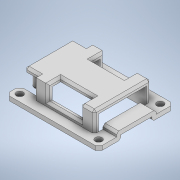
# Autodesk Inventor part: motor holder top
Saved by Autodesk Inventor 2022 (Build 260153000, 153)
## iProperties
Created: 2021-11-29
Part Number: motor holder top
Material: Generic
Document SubType Name: Modeling
Designer: Alec Warren
Density: 1 g/cm^3
Appearance: Default
Author: Alec Warren
Autodesk Inventor part; units mm, degrees
ref_plane "YZ Plane" through (0, 0, 0) normal (1, 0, 0) x (0, 1, 0)
ref_plane "XZ Plane" through (0, 0, 0) normal (0, 1, 0) x (-1, 0, 0)
ref_plane "XY Plane" through (0, 0, 0) normal (0, 0, 1) x (1, 0, 0)
sketch "Sketch1" plane through (0, 0, 0) normal (0, 1, 0) x (-1, 0, 0)
  line L0 (0, 0) -> (0, 22.5)
  line L1 (-41.8, 0) -> (0, 0)
  line L2 (0, 11.25) -> (-37, 11.25)
  line L3 (-39.4, 11.25) -> (-25.4, 11.25)
  line L4 (-25.4, 11.25) -> (-14.15, 11.25)
  line L5 (-14.15, 11.25) -> (-5.55, 11.25)
  line L6 (-5.55, 11.25) -> (-5.55, 2.45)
  line L7 (-5.55, 11.25) -> (-5.55, 20.05)
  circle A0 centre (-5.55, 2.45) radius 1.375
  circle A1 centre (-5.55, 20.05) radius 1.375
  line L8 (-37, 0) -> (-37, 22.5)
  line L9 (0, 22.5) -> (0, 28.9)
  line L10 (0, 0) -> (0, -6.4)
  line L11 (0, -6.4) -> (-41.8, -6.4)
  line L12 (-41.8, 28.9) -> (0, 28.9)
  line L13 (0, -3.2) -> (-3.2, -3.2)
  line L14 (0, 25.7) -> (-3.2, 25.7)
  circle A2 centre (-3.2, -3.2) radius 1.6
  circle A3 centre (-40.2, -3.2) radius 1.6
  circle A4 centre (-3.2, 25.7) radius 1.6
  circle A5 centre (-3.2, 25.7) radius 1.6
  circle A6 centre (-40.2, 25.7) radius 1.6
  line L15 (-5.55, 0) -> (-2.35, 0)
  line L16 (-5.55, 0) -> (-8.75, 0)
  line L17 (-2.35, 0) -> (-8.75, 0)
  line L18 (-8.75, 0) -> (-8.75, 22.5)
  line L19 (-8.75, 22.5) -> (-2.35, 22.5)
  line L20 (-2.35, 22.5) -> (-2.35, 0)
  line L21 (-37, 11.25) -> (-30.6, 11.25)
  line L22 (-30.6, 22.5) -> (-30.6, 0)
  line L23 (-37, 22.5) -> (-37, 28.9)
  line L24 (-30.6, 22.5) -> (-30.6, 28.9)
  line L25 (-30.6, 0) -> (-30.6, -6.4)
  line L26 (-37, -6.4) -> (-37, 0)
  line L27 (-8.75, 0) -> (-8.75, -6.4)
  line L28 (-8.75, 22.5) -> (-8.75, 28.9)
  line L29 (-37, 28.9) -> (-43.4, 28.9)
  line L30 (-43.4, 28.9) -> (-43.4, -6.4)
  line L31 (-43.4, -6.4) -> (-37, -6.4)
  line L32 (-8.75, 28.9) -> (-15.15, 28.9)
  line L33 (-15.15, 28.9) -> (-15.15, -6.4)
  line L34 (-30.6, 11.25) -> (-30.6, 22.5)
  line L35 (-30.6, 16.875) -> (-30.6, 18.475)
  line L36 (-30.6, 16.875) -> (-30.6, 15.275)
  line L37 (-30.6, 18.475) -> (-15.15, 18.475)
  line L38 (-15.15, 18.475) -> (-15.15, 15.275)
  line L39 (-30.6, 15.275) -> (-30.6, 18.475)
  line L40 (-43.4, 11.25) -> (-37, 11.25)
  line L41 (-30.6, 11.25) -> (-30.6, 0)
  line L42 (-30.6, 5.625) -> (-30.6, 4.025)
  line L43 (-30.6, 4.025) -> (-15.15, 4.025)
  line L44 (-37, 0) -> (-43.4, 0)
  line L45 (0, 28.9) -> (0, 22.5)
  line L46 (0, 22.5) -> (-43.4, 22.5)
  line L47 (0, 0) -> (-43.4, 0)
  line L48 (-37, 22.5) -> (-30.6, 22.5)
  line L49 (-30.6, 22.5) -> (-30.6, 24.5)
  line L50 (-30.6, 24.5) -> (-37, 24.5)
  line L51 (-37, 24.5) -> (-37, 22.5)
  line L52 (-37, 0) -> (-30.6, 0)
  line L53 (-30.6, 0) -> (-30.6, -2)
  line L54 (-30.6, -2) -> (-37, -2)
  line L55 (-37, -2) -> (-37, 0)
  line L56 (-15.15, 22.5) -> (-8.75, 22.5)
  line L57 (-8.75, 22.5) -> (-8.75, 24.5)
  line L58 (-8.75, 24.5) -> (-15.15, 24.5)
  line L59 (-15.15, 24.5) -> (-15.15, 22.5)
  line L60 (-15.15, 0) -> (-8.75, 0)
  line L61 (-8.75, 0) -> (-8.75, -2)
  line L62 (-8.75, -2) -> (-15.15, -2)
  line L63 (-15.15, -2) -> (-15.15, 0)
  line L64 (-30.6, 24.5) -> (-15.15, 24.5)
  line L65 (-15.15, -2) -> (-30.6, -2)
  line L66 (-37, 22.5) -> (-37, 18.5)
  line L67 (-37, 18.5) -> (-43.4, 18.5)
  line L68 (-37, 0) -> (-37, 4)
  line L69 (-37, 4) -> (-43.4, 4)
  line L70 (-43.4, 20.5) -> (-37, 20.5)
  line L71 (-37, 2) -> (-43.4, 2)
  point P0 (-15.15, 0)
  dimension "d0" = 22.5
  dimension "d2" = 37
  dimension "d4" = 14
  dimension "d5" = 11.25
  dimension "d6" = 8.6
  dimension "d7" = 8.8
  dimension "d8" = 8.8
  dimension "d9" = 2.75
  dimension "d10" = 2.75
  dimension "d12" = 6.4
  dimension "d13" = 6.4
  dimension "d18" = 3.2
  dimension "d22" = 3.2
  dimension "d39" = 3.2
  dimension "d40" = 3.2
  dimension "d41" = 6.4
  dimension "d42" = 6.4
  dimension "d43" = 6.4
  dimension "d44" = 1.6
  dimension "d45" = 1.6
  dimension "d46" = 1.6
  dimension "d47" = 2
  dimension "d48" = 2
  dimension "d49" = 2
  dimension "d50" = 2
  dimension "d57" = 4
  dimension "d58" = 4
  constraints: 142 end point, 37 point on line, 16 horizontal, 15 perpendicular, 14 parallel, 7 centre point, 7 midpoint, 5 collinear, 4 coincident, 4 vertical, 2 symmetric about line, 1 equal radius, 12 other
  measures "d0" distance of L0.start L0.end
  measures "d2" distance of L2.start L2.end
  measures "d4" distance of L3.start L3.end
  measures "d5" distance of L3.end L4.end
  measures "d6" distance of L4.end L5.end
  measures "d7" distance of L5.end L6.end
  measures "d8" distance of L5.end L7.end
  measures "d9" diameter of A0
  measures "d10" diameter of A1
  measures "d12" distance of L0.end L9.end
  measures "d13" distance of L0.start L10.end
  measures "d18" distance of L14.start L14.end
  measures "d22" diameter of A4
  measures "d39" distance of L15.start L15.end
  measures "d40" distance of L15.start L16.end
  measures "d41" distance of L2.end L21.end
  measures "d42" distance of L23.end L29.end
  measures "d43" distance of L28.end L32.end
  measures "d44" distance of L35.start L35.end
  measures "d45" distance of L35.start L36.end
  measures "d46" distance of L42.start L42.end
  measures "d47" distance of L49.end L48.end
  measures "d48" distance of L52.end L53.end
  measures "d49" distance of L57.end L56.end
  measures "d50" distance of L60.end L61.end
  measures "d57" distance of L8.end L66.end
  measures "d58" distance of L8.start L68.end
extrude "Extrusion1" add sketch "Sketch1" along normal blind 2 contours L10 L11 L27 L1 | L46 L19 L28 L12 L9 | L27 L62 L33 L1 | L11 L33 L62 L27 | L46 L33 L58 L28 | L33 L65 L25 L1 | L11 L25 L65 L33 | L28 L58 L33 L12 | L46 L24 L64 L33 | L25 L54 L26 L1 | L11 L26 L54 L25 | L33 L64 L24 L12 | L46 L23 L50 L24 | L26 L11 L31 L30 L44 L1 | L1 L44 L30 L71 L8 | L24 L50 L23 L12 | L46 L30 L29 L12 L23 | L8 L70 L30 L46 | L71 L30 L69 L8 | L8 L67 L30 L70
extrude "Extrusion5" add sketch "Sketch1" along normal blind 2 from surface at 2 contours L71 L30 L69 L8 | L8 L67 L30 L70 | L69 L30 L40 L3 L8 | L8 L3 L40 L30 L67
extrude "Extrusion6" add sketch "Sketch1" along normal blind 7.3 from surface at 2 contours L27 L62 L33 L1 | L46 L33 L58 L28 | L25 L54 L26 L1 | L46 L23 L50 L24
extrude "Extrusion7" add sketch "Sketch1" along normal blind 2 from surface at 9.3 contours L1 L18 L2 L20 | L2 L18 L19 L20 | L27 L62 L33 L1 | L1 L33 L2 L18 | L46 L33 L58 L28 | L18 L2 L33 L46 | L25 L54 L26 L1 | L1 L8 L2 L22 | L43 L22 L2 L33 | L33 L2 L22 L37 | L46 L23 L50 L24 | L22 L2 L8 L46 | A0 | A1
chamfer "Chamfer2" distance 1 angle 45 4 edges at (40.2, 0, 18.5) (40.2, 4, 20.5) (40.2, 4, 2) (40.2, 0, 4)
extrude "Extrusion8" add sketch "Sketch1" against normal blind 6.4 from surface at 9.3 contours A0 | A1
extrude "Extrusion9" add sketch "Sketch1" along normal blind 2 from surface at 2 contours L33 L65 L25 L1 | L46 L24 L64 L33
fillet "Fillet4" radius 1 2 edges at (6.925, 2.9, 20.05) (6.925, 2.9, 2.45)
chamfer "Chamfer3" distance 1 angle 45 26 edges at (5.55, 11.3, 22.5) (2.35, 11.3, 11.25) (5.55, 11.3, 0) (8.75, 11.3, -1) (33.8, 11.3, -2) (22.875, 11.3, 4.025) (15.15, 11.3, 21.4875) (15.15, 11.3, 1.0125) (22.875, 11.3, 18.475) (33.8, 11.3, 24.5) (8.75, 11.3, 23.5) (30.6, 11.3, 1.0125) (37, 11.3, 11.25) (30.6, 11.3, 21.4875) (15.15, 7.65, 24.5) (22.875, 4, 24.5) (30.6, 7.65, 24.5) (8.75, 6.65, 24.5) (8.75, 6.65, -2) (15.15, 7.65, -2) (30.6, 7.65, -2) (37, 6.65, -2) (22.875, 4, -2) (37, 6.65, 24.5) (2.35, 10.3, 0) (2.35, 10.3, 22.5)
chamfer "Chamfer4" distance 1.6 angle 45 6 edges at (0, 1, 28.9) (43.4, 1, 28.9) (43.4, 1, -6.4) (0, 1, -6.4) (0, 1, 0) (0, 1, 22.5)
body "Solid1"
